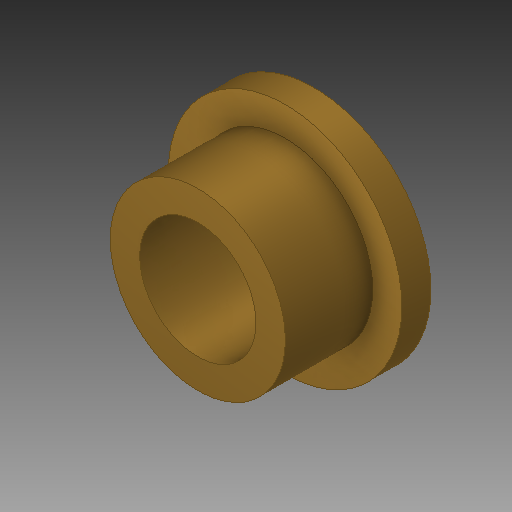
# Autodesk Inventor part: Flange Bearing
Saved by Autodesk Inventor 2017 (Build 210142000, 142)
## iProperties
Created: 2018-10-30
Part Number: Flange Bearing
Material: Brass, Soft Yellow
Document SubType Name: Modeling
Designer: Dell
Density: 8.47 g/cm^3
Appearance: Brass - Satin
Mass: 23.2621 g
Surface Area: 21.0116 cm^2
Volume: 2.74641 cm^3
Author: Dell
Autodesk Inventor part; units mm, degrees
ref_plane "YZ Plane" through (0, 0, 0) normal (1, 0, 0) x (0, 1, 0)
ref_plane "XZ Plane" through (0, 0, 0) normal (0, 1, 0) x (-1, 0, 0)
ref_plane "XY Plane" through (0, 0, 0) normal (0, 0, 1) x (1, 0, 0)
sketch "Sketch1" plane through (0, 0, 0) normal (0, 0, 1) x (1, 0, 0)
  circle A0 centre (0, 0) radius 9.56
  circle A1 centre (0, 0) radius 6.35
  dimension "d0" = 19.12
  dimension "d1" = 12.7
  constraints: 2 centre point, 2 coincident
  measures "d0" diameter of A0
  measures "d1" diameter of A1
extrude "Extrusion1" add sketch "Sketch1" along normal blind 12.7
sketch "Sketch2" plane through (0, 0, 0) normal (0, 0, -1) x (-1, 0, 0)
  circle A0 centre (0, 0) radius 12.75
  circle A1 centre (0, 0) radius 9.56 projected
  dimension "d4" = 25.5
  constraints: 1 centre point, 1 coincident
  measures "d4" diameter of A0
extrude "Extrusion2" add sketch "Sketch2" against normal blind 3.17
body "Solid1"
